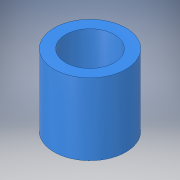
# Autodesk Inventor part: Idle_pulley_small
Saved by Autodesk Inventor 2019.4 (Build 234330000, 330)
## iProperties
Created: 2021-02-03
Part Number: Idle_pulley_small
Material: Generic
Document SubType Name: Modeling
Designer: Jorian Brusind
Density: 1 g/cm^3
Appearance: Cyan
Author: Jorian Brusind
Autodesk Inventor part; units mm, degrees
ref_plane "YZ Plane" through (0, 0, 0) normal (1, 0, 0) x (0, 1, 0)
ref_plane "XZ Plane" through (0, 0, 0) normal (0, 1, 0) x (-1, 0, 0)
ref_plane "XY Plane" through (0, 0, 0) normal (0, 0, 1) x (1, 0, 0)
sketch "Sketch1" plane through (0, 0, 0) normal (0, 1, 0) x (-1, 0, 0)
  circle A0 centre (0, 0) radius 4.75
  line L0 (0, 0) -> (15.4998, -15.4998)
  line L1 (0, 0) -> (21.92, 0) construction
  circle A1 centre (15.4998, -15.4998) radius 10.75
  circle A2 centre (0, 0) radius 7
  dimension "d0" = 9.5
  dimension "d1" = 21.92
  dimension "d2" = 45
  dimension "d3" = 21.5
  dimension "d4" = 14
  constraints: 4 end point, 3 centre point, 3 coincident, 1 equal length, 1 horizontal
  measures "d0" diameter of A0
  measures "d1" distance of L0.start L0.end
  measures "d2" angle of L0 L1
  measures "d3" diameter of A1
  measures "d4" diameter of A2
extrude "Extrusion1" add sketch "Sketch1" along normal blind 14 contours A2
body "Solid1"
